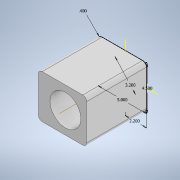
# Autodesk Inventor part: cylinder
Saved by Autodesk Inventor 2021.1 (Build 251245000, 245)
## iProperties
Created: 2020-08-30
Part Number: cylinder
Material: Generic
Document SubType Name: Sheet Metal
Designer: Vamshi
Density: 1 g/cm^3
Sheet Metal Rule: Default
Appearance: Default
Author: Vamshi
Autodesk Inventor part; units mm, degrees
ref_plane "YZ Plane" through (0, 0, 0) normal (1, 0, 0) x (0, 1, 0)
ref_plane "XZ Plane" through (0, 0, 0) normal (0, 1, 0) x (-1, 0, 0)
ref_plane "XY Plane" through (0, 0, 0) normal (0, 0, 1) x (1, 0, 0)
sketch "Sketch1" plane through (0, 0, 0) normal (0, 0, 1) x (1, 0, 0)
  line L0 (-60.96, 57.15) -> (45.72, 57.15)
  line L1 (55.88, 46.99) -> (55.88, -46.99)
  line L2 (45.72, -57.15) -> (-60.96, -57.15)
  line L3 (-71.12, -46.99) -> (-71.12, 46.99)
  line L4 (-99.4659, 0) -> (84.2259, 0) projected
  line L5 (0, -82.9559) -> (0, 82.9559) projected
  arc A0 (-60.96, 57.15) -> (-71.12, 46.99) centre (-60.96, 46.99) ccw
  arc A1 (55.88, 46.99) -> (45.72, 57.15) centre (45.72, 46.99) ccw
  arc A2 (45.72, -57.15) -> (55.88, -46.99) centre (45.72, -46.99) ccw
  arc A3 (-71.12, -46.99) -> (-60.96, -57.15) centre (-60.96, -46.99) ccw
  circle A4 centre (0, 0) radius 40.64
  point P0 (55.88, -57.15)
  point P1 (55.88, 57.15)
  point P2 (-71.12, -57.15)
  point P3 (-71.12, 0)
  dimension "d0" = 127
  dimension "d1" = 114.3
  dimension "d2" = 55.88
  dimension "d3" = 10.16
  dimension "d6" = 81.28
  constraints: 8 end point, 8 point on circle, 8 tangent, 7 point on line, 5 centre point, 3 equal radius, 2 parallel, 1 coincident, 1 horizontal, 1 midpoint, 1 perpendicular
  measures "d0" distance of point (55.88, -57.15) point (-71.12, -57.15)
  measures "d1" distance of point (55.88, 57.15) point (55.88, -57.15)
  measures "d2" distance between parallel lines of L5 L1
  measures "d3" radius of A0
  measures "d6" diameter of A4
extrude "Extrusion1" add sketch "Sketch1" along normal blind 157.48
extrude "Extrusion2" cut sketch "Sketch1" along normal blind 157.48 contours A4 L4 L5 | L5 L4 A4 | L5 A4 L4 | L4 A4 L5
equation "\"BendRadius\" = Thickness"
equation "\"BendReliefWidth\" = Thickness"
equation "\"BendReliefDepth\" = 0.5 * Thickness"
equation "\"CornerReliefSize\" = 4 * Thickness"
equation "\"MinimumRemnant\" = 2 * Thickness"
equation "\"TransitionRadius\" = BendRadius"
equation "\"JacobiRadiusSize\" = BendRadius"
equation "\"GapSize\" = Thickness"
equation "\"Thickness\" = 3.048"
body "Solid1"
